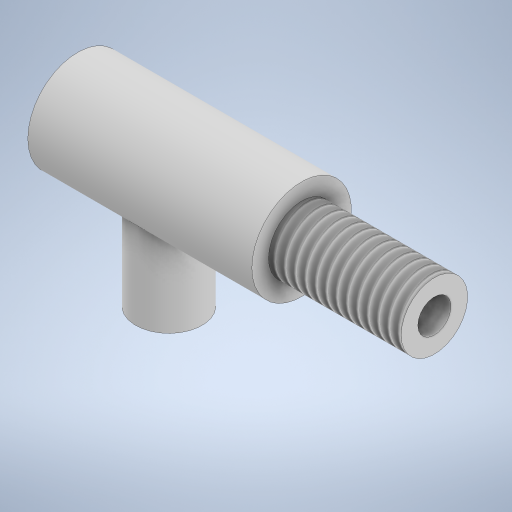
# Autodesk Inventor part: HUDSON-1-81
Saved by Autodesk Inventor 2024.2 (Build 282272000, 272)
## iProperties
Created: 2024-10-05
Part Number: HUDSON-1-81
Material: Generic
Document SubType Name: Modeling
Designer: melim
Density: 1 g/cm^3
Appearance: Default
Author: melim
Autodesk Inventor part; units mm, degrees
note: some values were not read from the file. Chosen so that the rebuilt part matches the saved one: direction of "Hole2".
ref_plane "YZ Plane" through (0, 0, 0) normal (1, 0, 0) x (0, 1, 0)
ref_plane "XY Plane" through (0, 0, 0) normal (0, 0, 1) x (1, 0, 0)
sketch "Sketch1" plane through (0, 0, 0) normal (0, 1, 0) x (-1, 0, 0)
  line L0 (0, 0) -> (-52, 0)
  line L1 (0, 4) -> (-8, 4)
  line L2 (0, 6) -> (-27, 6)
  line L3 (0, 0) -> (0, 37) construction
  line L4 (-8, 3.25) -> (-20, 3.25)
  line L5 (-8, 4) -> (-8, 3.25)
  line L6 (-20, 1.5) -> (-27, 1.5)
  line L7 (-20, 3.25) -> (-20, 1.5)
  line L8 (-27, 6) -> (-27, 4)
  line L9 (-27, 4) -> (-43, 4)
  line L10 (-34, 2) -> (-43, 2)
  line L11 (-43, 4) -> (-43, 2)
  line L12 (-34, 2) -> (-34, 1.5)
  line L13 (-34, 1.5) -> (-27, 1.5)
  line L14 (0, 6) -> (0, 4)
  point P0 (-8, 3.625)
  dimension "d0" = 8
  dimension "d1" = 12
  dimension "d2" = 27
  dimension "d3" = 6.5
  dimension "d4" = 8
  dimension "d5" = 20
  dimension "d6" = 3
  dimension "d7" = 8
  dimension "d8" = 16
  dimension "d9" = 4
  dimension "d10" = 9
  constraints: 30 end point, 6 horizontal, 4 vertical, 3 perpendicular, 1 collinear, 1 midpoint, 1 point on line
  measures "d0" diameter of L1 L0
  measures "d1" diameter of L2 L0
  measures "d2" distance of L2.start L2.end
  measures "d3" diameter of L4.end L0
  measures "d4" distance from line of L3 point (-8, 3.625)
  measures "d5" distance from line of L3 L4.end
  measures "d6" diameter of L6 L0
  measures "d7" diameter of L9 L0
  measures "d8" distance of L8.end L9.end
  measures "d9" diameter of L10 L0
  measures "d10" distance of L10.start L10.end
revolve "Revolution1" add sketch "Sketch1" angle 360 about axis through (0, 0, 0) along (1, 0, 0)
thread "Thread1" size "M8x1.25" class "6g" standard "ANSI Metric M Profile" full length
thread "Thread2" size "M8x1.25" class "6H" standard "ANSI Metric M Profile" full length
ref_plane "Work Plane1" through (13.5, -6, 0) normal (0, 1, 0) x (-1, 0, 0)
sketch "Sketch2" plane through (13.5, -6, 0) normal (0, 1, 0) x (-1, 0, 0)
  circle A0 centre (2.5, 0) radius 4
  line L0 (13.5, 6) -> (13.5, -6) projected
  line L1 (13.5, 0) -> (-13.5, 0)
  line L2 (-13.5, 6) -> (-13.5, -6) projected
  dimension "d16" = 8
  dimension "d17" = 7
  constraints: 2 end point, 1 centre point, 1 midpoint, 1 point on line
  measures "d16" diameter of A0
  measures "d17" distance edge to line of A0 L0
extrude "Extrusion1" add sketch "Sketch2" against normal blind 9
sketch "Sketch3" plane through (11, -15, 0) normal (0, -1, 0) x (1, 0, 0)
  circle A0 centre (0, 0) radius 4 projected
  point P0 (-11, 0)
extrude "Extrusion2" add sketch "Sketch2" along normal blind 2
hole "Hole2" at (11, -15, 0) direction (0, 1, 0) diameter 4 end up to surface
body "Solid1"
